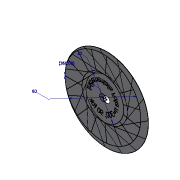
# Autodesk Inventor part: InkrementalisFolia
Saved by Autodesk Inventor 2015 SP1 (Build 190203100, 203)
## iProperties
Created: 2014-11-14
Part Number: InkrementalisFolia
Material: Generic
Document SubType Name: Modeling
Designer: laca
Density: 1 g/cm^3
Appearance: Default
Mass: 0.340156 g
Surface Area: 68.2542 cm^2
Volume: 0.340156 cm^3
d32: 360.00 deg
Author: laca
Autodesk Inventor part; units mm, degrees
ref_plane "YZ Plane" through (0, 0, 0) normal (1, 0, 0) x (0, 1, 0)
ref_plane "XZ Plane" through (0, 0, 0) normal (0, 1, 0) x (-1, 0, 0)
ref_plane "XY Plane" through (0, 0, 0) normal (0, 0, 1) x (1, 0, 0)
sketch "Sketch1" plane through (0, 0, 0) normal (0, 1, 0) x (-1, 0, 0)
  circle A0 centre (0, 0) radius 32.5
  circle A1 centre (0, 0) radius 22.5
  circle A2 centre (0, 0) radius 16
  line L0 (22.5, 0) -> (32.5, 0)
  point P0 (32.4988, -0.2836)
  point P1 (22.4991, -0.1963)
  dimension "d0" = 65
  dimension "d2" = 10
  dimension "d3" = 32
  constraints: 4 point on circle, 3 centre point, 3 coincident, 2 end point, 1 horizontal
  measures "d0" diameter of A0
  measures "d2" radial gap between concentric circles of A0 A1
  measures "d3" diameter of A2
extrude "Extrusion1" [suppressed]
extrude "Extrusion2" [suppressed]
pattern_circular "Circular Pattern1" [suppressed]
sketch "Sketch3" plane through (0, 0, 0) normal (0, 0, 1) x (1, 0, 0)
  circle A0 centre (0, 0) radius 33
  circle A1 centre (0, 0) radius 16.5
  circle A2 centre (0, 0) radius 2.5
  line L0 (-13.516, 9.464) -> (-31.7996, -8.8196)
  line L1 (0, 0) -> (-2.5, 0)
  line L2 (-16.1968, 3.1483) -> (-25.4631, -20.9912)
  line L3 (-16.0771, -3.7117) -> (-14.7239, -29.5332)
  line L4 (-13.1775, -9.9299) -> (-1.4387, -32.9686)
  line L5 (-7.9994, -14.4312) -> (12.0952, -30.7035)
  line L6 (-1.4381, -16.4372) -> (23.5378, -23.1295)
  line L7 (5.3719, -15.6011) -> (30.9104, -11.5561)
  line L8 (11.253, -12.0673) -> (32.9384, 2.0153)
  line L9 (15.1883, -6.4471) -> (29.271, 15.2384)
  line L10 (16.4975, 0.288) -> (20.5424, 25.8265)
  line L11 (14.9541, 6.9732) -> (8.2618, 31.9491)
  line L12 (10.825, 12.4527) -> (-5.4473, 32.5473)
  line L13 (4.8241, 15.779) -> (-18.2145, 27.5178)
  line L14 (-2.0108, 16.377) -> (-27.8323, 17.7303)
  line L15 (-8.4981, 14.1433) -> (-32.6376, 4.877)
  dimension "d21" = 66
  dimension "d27" = 33
  dimension "d28" = 5
  dimension "d29" = 45
  dimension "d32" = 360
  constraints: 32 end point, 3 coincident, 1 horizontal, 1 horizontal alignment, 54 other
  measures "d29" angle of L0 L1
extrude "Extrusion6" add sketch "Sketch3" along normal blind 0.1
sketch "Sketch4" plane through (0, 0, 0.1) normal (0, 0, 1) x (1, 0, 0)
  circle A0 centre (-3, -0.0066) radius 30
  circle A1 centre (-3, -0.0066) radius 16.5
  circle A2 centre (-3, -0.0066) radius 2.5
  line L0 (-3, -0.0066) -> (-5.5, -0.0066)
  circle A3 centre (0, 0) radius 33 projected
  line L1 (-32.9999, 0.0596) -> (-19.4999, 0.0596)
  line L2 (-30.4332, -12.1482) -> (-18.1003, -6.6573)
  line L3 (-23.1231, -22.2566) -> (-14.0898, -12.2241)
  line L4 (-12.3335, -28.5178) -> (-8.1617, -15.6785)
  line L5 (0.07, -29.8491) -> (-1.3411, -16.423)
  line L6 (11.9426, -26.0204) -> (5.1926, -14.329)
  line L7 (21.2315, -17.6937) -> (10.3098, -9.7585)
  line L8 (26.3306, -6.3087) -> (13.1255, -3.5019)
  line L9 (26.3581, 6.166) -> (13.153, 3.3592)
  line L10 (21.3093, 17.5734) -> (10.3876, 9.6382)
  line L11 (12.0573, 25.941) -> (5.3072, 14.2496)
  line L12 (0.2016, 29.822) -> (-1.2095, 16.3959)
  line L13 (-12.2076, 28.5455) -> (-8.0358, 15.7061)
  line L14 (-23.0247, 22.332) -> (-13.9914, 12.2995)
  line L15 (-30.3794, 12.2559) -> (-18.0465, 6.7649)
  dimension "d44" = 60
  dimension "d45" = 33
  dimension "d46" = 5
  dimension "d51" = 360
  constraints: 32 end point, 3 coincident, 2 horizontal, 1 horizontal alignment, 56 other
body "Solid1"
